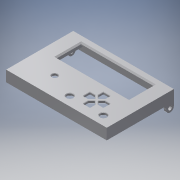
# Autodesk Inventor part: Interface Frame
Saved by Autodesk Inventor 2018 (Build 220112000, 112)
## iProperties
Created: 2018-03-12
Part Number: Interface Frame
Material: ABS Plastic
Document SubType Name: Modeling
Designer: Gabriel Smolnycki
Density: 1.06 g/cm^3
Appearance: Smooth - White
Author: Gabriel Smolnycki
Autodesk Inventor part; units mm, degrees
ref_plane "YZ Plane" through (0, 0, 0) normal (1, 0, 0) x (0, 1, 0)
ref_plane "XZ Plane" through (0, 0, 0) normal (0, 1, 0) x (-1, 0, 0)
sketch "Sketch1" plane through (0, 0, 0) normal (0, 0, 1) x (1, 0, 0)
  line L0 (-60, -40) -> (60, -40)
  line L1 (60, -40) -> (60, 40)
  line L2 (60, 40) -> (-60, 40)
  line L3 (-60, 40) -> (-60, -40)
  line L4 (-60, -40) -> (60, 40) construction
  line L5 (60, -40) -> (-60, 40) construction
  point P0 (0, 0)
  dimension "d0" = 120
  dimension "d1" = 80
  constraints: 12 end point, 2 midpoint, 2 parallel, 1 horizontal, 1 perpendicular
  measures "d0" distance of L2.end L1.end
  measures "d1" distance of L1.end L0.end
extrude "Extrusion1" add sketch "Sketch1" against normal blind 3
sketch "Sketch2" plane through (0, 0, 0) normal (0, 0, 1) x (1, 0, 0)
  line L0 (-43, 32.5) -> (43, 32.5)
  line L1 (43, 32.5) -> (43, 3.5)
  line L2 (43, 3.5) -> (-43, 3.5)
  line L3 (-43, 3.5) -> (-43, 32.5)
  line L4 (-43, 32.5) -> (43, 3.5) construction
  line L5 (43, 32.5) -> (-43, 3.5) construction
  point P0 (0, 0)
  point P1 (0, 18)
  dimension "d4" = 86
  dimension "d5" = 29
  dimension "d6" = 18
  constraints: 12 end point, 2 midpoint, 2 parallel, 1 horizontal, 1 perpendicular
  measures "d4" distance of L1.end L2.end
  measures "d5" distance of L0.end L1.end
  measures "d6" distance of point (0, 0) point (0, 18)
extrude "Extrusion2" cut sketch "Sketch2" against normal through all
chamfer "Chamfer1" distance 1.5 angle 45 4 edges at (-43, 18, 0) (0, 32.5, 0) (43, 18, 0) (0, 3.5, 0)
sketch "Sketch3" plane through (0, 0, 0) normal (0, 0, 1) x (1, 0, 0)
  line L0 (28.5, -29) -> (21.5, -29)
  line L1 (21, -28.5) -> (21, -23.2071)
  line L2 (29, -23.2071) -> (29, -28.5)
  line L3 (21.1464, -22.8536) -> (24.6464, -19.3536)
  line L4 (25.3536, -19.3536) -> (28.8536, -22.8536)
  arc A0 (21.1464, -22.8536) -> (21, -23.2071) centre (21.5, -23.2071) ccw
  arc A1 (21, -28.5) -> (21.5, -29) centre (21.5, -28.5) ccw
  arc A2 (28.5, -29) -> (29, -28.5) centre (28.5, -28.5) ccw
  arc A3 (29, -23.2071) -> (28.8536, -22.8536) centre (28.5, -23.2071) ccw
  arc A4 (25.3536, -19.3536) -> (24.6464, -19.3536) centre (25, -19.7071) ccw
  line L5 (60, -40) -> (60, 40) projected
  line L6 (-60, -40) -> (60, -40) projected
  line L7 (0, 0) -> (60, 0) construction
  line L8 (0, 0) -> (0, -40) construction
  line L9 (60, -40) -> (-60, -40) construction
  arc A5 (31.2071, -13) -> (30.8536, -13.1464) centre (31.2071, -13.5) ccw
  line L10 (31.2071, -13) -> (36.5, -13)
  arc A6 (27.3536, -16.6464) -> (27.3536, -17.3536) centre (27.7071, -17) ccw
  arc A7 (37, -13.5) -> (36.5, -13) centre (36.5, -13.5) ccw
  arc A8 (30.8536, -20.8536) -> (31.2071, -21) centre (31.2071, -20.5) ccw
  line L11 (30.8536, -20.8536) -> (27.3536, -17.3536)
  line L12 (36.5, -21) -> (31.2071, -21)
  arc A9 (36.5, -21) -> (37, -20.5) centre (36.5, -20.5) ccw
  line L13 (37, -13.5) -> (37, -20.5)
  line L14 (27.3536, -16.6464) -> (30.8536, -13.1464)
  arc A10 (21, -10.7929) -> (21.1464, -11.1464) centre (21.5, -10.7929) ccw
  line L15 (21, -10.7929) -> (21, -5.5)
  arc A11 (24.6464, -14.6464) -> (25.3536, -14.6464) centre (25, -14.2929) ccw
  arc A12 (21.5, -5) -> (21, -5.5) centre (21.5, -5.5) ccw
  arc A13 (28.8536, -11.1464) -> (29, -10.7929) centre (28.5, -10.7929) ccw
  line L16 (28.8536, -11.1464) -> (25.3536, -14.6464)
  line L17 (29, -5.5) -> (29, -10.7929)
  arc A14 (29, -5.5) -> (28.5, -5) centre (28.5, -5.5) ccw
  line L18 (21.5, -5) -> (28.5, -5)
  line L19 (24.6464, -14.6464) -> (21.1464, -11.1464)
  arc A15 (18.7929, -21) -> (19.1464, -20.8536) centre (18.7929, -20.5) ccw
  line L20 (18.7929, -21) -> (13.5, -21)
  arc A16 (22.6464, -17.3536) -> (22.6464, -16.6464) centre (22.2929, -17) ccw
  arc A17 (13, -20.5) -> (13.5, -21) centre (13.5, -20.5) ccw
  arc A18 (19.1464, -13.1464) -> (18.7929, -13) centre (18.7929, -13.5) ccw
  line L21 (19.1464, -13.1464) -> (22.6464, -16.6464)
  line L22 (13.5, -13) -> (18.7929, -13)
  arc A19 (13.5, -13) -> (13, -13.5) centre (13.5, -13.5) ccw
  line L23 (13, -20.5) -> (13, -13.5)
  line L24 (22.6464, -17.3536) -> (19.1464, -20.8536)
  circle A20 centre (45, -29) radius 4
  circle A21 centre (5, -29) radius 4
  circle A22 centre (-25, -17) radius 3.25
  point P0 (29, -29)
  point P1 (21, -29)
  point P2 (21, -23)
  point P3 (29, -23)
  point P4 (25, -19)
  point P5 (25, -17)
  point P6 (37, -13)
  point P7 (31, -13)
  point P8 (27, -17)
  point P9 (31, -21)
  point P10 (37, -21)
  point P11 (21, -5)
  point P12 (21, -11)
  point P13 (25, -15)
  point P14 (29, -11)
  point P15 (29, -5)
  point P16 (13, -21)
  point P17 (19, -21)
  point P18 (23, -17)
  point P19 (19, -13)
  point P20 (13, -13)
  dimension "d13" = 8
  dimension "d18" = 45
  dimension "d19" = 45
  dimension "d20" = 10
  dimension "d21" = 6
  dimension "d22" = 0.5
  dimension "d23" = 40
  dimension "d24" = 60
  dimension "d25" = 25
  dimension "d26" = 17
  dimension "d29" = 360
  dimension "d31" = 2
  dimension "d32" = 8
  dimension "d33" = 8
  dimension "d38" = 20
  dimension "d39" = 20
  dimension "d40" = 6.5
  dimension "d41" = 25
  dimension "d42" = 17
  dimension "d45" = 12
  dimension "d46" = 12
  constraints: 44 end point, 40 point on circle, 40 point on line, 23 centre point, 10 tangent, 4 equal radius, 2 midpoint, 2 perpendicular, 1 horizontal alignment, 1 vertical, 1 vertical alignment, 121 other
  measures "d13" distance of point (29, -29) point (21, -29)
  measures "d18" angle of L1 L3
  measures "d19" angle of L2 L4
  measures "d20" distance from line of L0 point (25, -19)
  measures "d21" distance of point (29, -29) point (29, -23)
  measures "d22" radius of A0
  measures "d23" distance of L7.start L8.end
  measures "d24" distance of L7.start L7.end
  measures "d25" distance from line of point (25, -17) L8
  measures "d26" distance from line of L7 point (25, -17)
  measures "d31" distance of point (25, -17) point (25, -19)
  measures "d32" diameter of A20
  measures "d33" diameter of A21
  measures "d38" horizontal distance of A20.centre point (25, -17)
  measures "d39" horizontal distance of A21.centre point (25, -17)
  measures "d40" diameter of A22
  measures "d41" distance from line of A22.centre L8
  measures "d42" vertical distance of L7.start A22.centre
  measures "d45" vertical distance of A21.centre point (25, -17)
  measures "d46" vertical distance of A20.centre point (25, -17)
extrude "Extrusion3" cut sketch "Sketch3" against normal through all
sketch "Sketch4" plane through (0, 0, -3) normal (0, 0, -1) x (-1, 0, 0)
  line L0 (60, -40) -> (60, 40) projected
  line L1 (-60, -40) -> (60, -40)
  line L2 (60, -40) -> (60, 40)
  line L3 (60, 40) -> (-60, 40)
  line L4 (-60, 40) -> (-60, -40)
  line L5 (-60, -40) -> (60, 40) construction
  line L6 (60, -40) -> (-60, 40) construction
  line L7 (-57, 37) -> (57, 37)
  line L8 (57, 37) -> (57, -37)
  line L9 (57, -37) -> (-57, -37)
  line L10 (-57, -37) -> (-57, 37)
  point P0 (0, 0)
  dimension "d47" = 3
  constraints: 20 end point, 4 parallel, 2 midpoint, 2 perpendicular, 1 horizontal, 3 other
  measures "d47" distance between parallel lines of L3 L7
extrude "Extrusion4" add sketch "Sketch4" along normal blind 10
sketch "Sketch5" plane through (60, -40, 0) normal (1, 0, 0) x (0, 0, -1)
  line L0 (13, 80) -> (13, 0) projected
  line L1 (0, 80) -> (13, 80) projected
  line L2 (0, 0) -> (0, 80) projected
  line L3 (13, 80) -> (13, 71)
  line L4 (13, 80) -> (17.5, 80)
  line L5 (17.5, 80) -> (17.5, 71) construction
  line L6 (17.5, 71) -> (13, 71)
  arc A0 (17.5, 71) -> (17.5, 80) centre (17.5, 75.5) ccw
  circle A1 centre (17.5, 75.5) radius 2.25
  point P0 (0, 40)
  dimension "d60" = 4.5
  dimension "d61" = 9
  dimension "d62" = 4.5
  dimension "d63" = 4.5
  constraints: 8 end point, 2 centre point, 2 perpendicular, 2 point on circle, 1 coincident, 1 horizontal, 1 point on line
  measures "d60" distance of L0.start L4.end
  measures "d61" distance of L0.start L3.end
  measures "d62" radius of A0
  measures "d63" diameter of A1
extrude "Extrusion5" add sketch "Sketch5" against normal up to surface (3 mm away)
mirror "Mirror1" about plane through (0, 0, 0) normal (1, 0, 0) of "Extrusion5"
fillet "Fillet2" radius 3 4 edges at (-57, 38.5, -13) (57, 38.5, -13) (58.5, 31, -13) (-58.5, 31, -13)
chamfer "Chamfer2" distance 0.5 angle 45 86 edges at (-28.25, -17, 0) (1, -29, 0) (21, -25.8536, 0) (21.0381, -23.0158, 0) (22.8964, -21.1036, 0) (25, -19.2071, 0) (27.1036, -21.1036, 0) (28.9619, -23.0158, 0) (29, -25.8536, 0) (28.8536, -28.8536, 0) (25, -29, 0) (21.1464, -28.8536, 0) (20.8964, -19.1036, 0) (18.9842, -20.9619, 0) (16.1464, -21, 0) (13.1464, -20.8536, 0) (13, -17, 0) (13.1464, -13.1464, 0) (16.1464, -13, 0) (18.9842, -13.0381, 0) (20.8964, -14.8964, 0) (22.7929, -17, 0) (25, -14.7929, 0) (22.8964, -12.8964, 0) (21.0381, -10.9842, 0) (21, -8.1464, 0) (21.1464, -5.1464, 0) (25, -5, 0) (28.8536, -5.1464, 0) (29, -8.1464, 0) (28.9619, -10.9842, 0) (27.1036, -12.8964, 0) (33.8536, -13, 0) (36.8536, -13.1464, 0) (37, -17, 0) (36.8536, -20.8536, 0) (33.8536, -21, 0) (31.0158, -20.9619, 0) (29.1036, -19.1036, 0) (27.2071, -17, 0) (29.1036, -14.8964, 0) (31.0158, -13.0381, 0) (41, -29, 0) (-28.25, -17, -3) (13, -17, -3) (13.1464, -20.8536, -3) (16.1464, -21, -3) (18.9842, -20.9619, -3) (20.8964, -19.1036, -3) (22.7929, -17, -3) (20.8964, -14.8964, -3) (18.9842, -13.0381, -3) (16.1464, -13, -3) (13.1464, -13.1464, -3) (1, -29, -3) (41, -29, -3) (25, -19.2071, -3) (22.8964, -21.1036, -3) (21.0381, -23.0158, -3) (21, -25.8536, -3) (21.1464, -28.8536, -3) (25, -29, -3) (28.8536, -28.8536, -3) (29, -25.8536, -3) (28.9619, -23.0158, -3) (27.1036, -21.1036, -3) (22.8964, -12.8964, -3) (25, -14.7929, -3) (27.1036, -12.8964, -3) (28.9619, -10.9842, -3) (29, -8.1464, -3) (28.8536, -5.1464, -3) (25, -5, -3) (21.1464, -5.1464, -3) (21, -8.1464, -3) (21.0381, -10.9842, -3) (29.1036, -14.8964, -3) (27.2071, -17, -3) (29.1036, -19.1036, -3) (31.0158, -20.9619, -3) (33.8536, -21, -3) (36.8536, -20.8536, -3) (37, -17, -3) (36.8536, -13.1464, -3) (33.8536, -13, -3) (31.0158, -13.0381, -3)
sketch "Sketch6" plane through (0, 0, -3) normal (0, 0, -1) x (-1, 0, 0)
  line L0 (-42.75, 3.75) -> (-46.75, 3.75) projected
  line L1 (-42.75, 4.25) -> (-42.75, 3.75) projected
  line L2 (42.75, 4.25) -> (-42.75, 4.25) projected
  line L3 (42.75, 3.75) -> (42.75, 4.25) projected
  line L4 (45.25, 3.75) -> (42.75, 3.75) projected
  line L5 (45.25, 5.5) -> (45.25, 3.75) projected
  line L6 (44.95, 5.5) -> (45.25, 5.5) projected
  arc A0 (44.95, 8) -> (44.95, 5.5) centre (44.95, 6.75) ccw projected
  line L7 (45.25, 8) -> (44.95, 8) projected
  line L8 (45.25, 31) -> (45.25, 8) projected
  line L9 (44.95, 31) -> (45.25, 31) projected
  arc A1 (44.95, 33.5) -> (44.95, 31) centre (44.95, 32.25) ccw projected
  line L10 (45.25, 33.5) -> (44.95, 33.5) projected
  line L11 (45.25, 35.25) -> (45.25, 33.5) projected
  line L12 (-46.75, 35.25) -> (45.25, 35.25) projected
  line L13 (-46.75, 33.5) -> (-46.75, 35.25) projected
  line L14 (-46.45, 33.5) -> (-46.75, 33.5) projected
  arc A2 (-46.45, 31) -> (-46.45, 33.5) centre (-46.45, 32.25) ccw projected
  line L15 (-46.75, 31) -> (-46.45, 31) projected
  line L16 (-46.75, 23.3) -> (-46.75, 31) projected
  line L17 (-43.75, 23.3) -> (-46.75, 23.3) projected
  arc A3 (-43.25, 22.8) -> (-43.75, 23.3) centre (-43.75, 22.8) ccw projected
  line L18 (-43.25, 13.3) -> (-43.25, 22.8) projected
  arc A4 (-43.75, 12.8) -> (-43.25, 13.3) centre (-43.75, 13.3) ccw projected
  line L19 (-46.75, 12.8) -> (-43.75, 12.8) projected
  line L20 (-46.75, 8) -> (-46.75, 12.8) projected
  line L21 (-46.45, 8) -> (-46.75, 8) projected
  arc A5 (-46.45, 5.5) -> (-46.45, 8) centre (-46.45, 6.75) ccw projected
  line L22 (-46.75, 5.5) -> (-46.45, 5.5) projected
  line L23 (-46.75, 3.75) -> (-46.75, 5.5) projected
  circle A6 centre (23.38, 33.75) radius 0.5 projected
  circle A7 centre (20.84, 33.75) radius 0.5 projected
  circle A8 centre (18.3, 33.75) radius 0.5 projected
  circle A9 centre (15.76, 33.75) radius 0.5 projected
  circle A10 centre (13.22, 33.75) radius 0.5 projected
  circle A11 centre (10.68, 33.75) radius 0.5 projected
  circle A12 centre (8.14, 33.75) radius 0.5 projected
  circle A13 centre (5.6, 33.75) radius 0.5 projected
  circle A14 centre (3.06, 33.75) radius 0.5 projected
  circle A15 centre (0.52, 33.75) radius 0.5 projected
  circle A16 centre (-2.02, 33.75) radius 0.5 projected
  circle A17 centre (-4.56, 33.75) radius 0.5 projected
  circle A18 centre (-7.1, 33.75) radius 0.5 projected
  circle A19 centre (-9.64, 33.75) radius 0.5 projected
  circle A20 centre (-12.18, 33.75) radius 0.5 projected
  circle A21 centre (-14.72, 33.75) radius 0.5 projected
  circle A22 centre (-17.26, 33.75) radius 0.5 projected
  circle A23 centre (-19.8, 33.75) radius 0.5 projected
  circle A24 centre (-22.34, 33.75) radius 0.5 projected
  circle A25 centre (-24.88, 33.75) radius 0.5 projected
  arc A26 (30.75, 32.3) -> (30.5, 32.55) centre (30.5, 32.3) ccw projected
  line L24 (30.75, 32.3) -> (30.75, 32) projected
  arc A27 (30.5, 31.75) -> (30.75, 32) centre (30.5, 32) ccw projected
  line L25 (30.5, 31.75) -> (26.5, 31.75) projected
  arc A28 (26.25, 32) -> (26.5, 31.75) centre (26.5, 32) ccw projected
  line L26 (26.25, 32) -> (26.25, 32.3) projected
  arc A29 (26.5, 32.55) -> (26.25, 32.3) centre (26.5, 32.3) ccw projected
  line L27 (26.5, 32.55) -> (30.5, 32.55) projected
  arc A30 (-27.75, 32.3) -> (-28, 32.55) centre (-28, 32.3) ccw projected
  line L28 (-27.75, 32.3) -> (-27.75, 32) projected
  arc A31 (-28, 31.75) -> (-27.75, 32) centre (-28, 32) ccw projected
  line L29 (-28, 31.75) -> (-32, 31.75) projected
  arc A32 (-32.25, 32) -> (-32, 31.75) centre (-32, 32) ccw projected
  line L30 (-32.25, 32) -> (-32.25, 32.3) projected
  arc A33 (-32, 32.55) -> (-32.25, 32.3) centre (-32, 32.3) ccw projected
  line L31 (-32, 32.55) -> (-28, 32.55) projected
  line L32 (-24.2929, -15) -> (-20.7929, -11.5) projected
  arc A34 (-25.7071, -15) -> (-24.2929, -15) centre (-25, -14.2929) ccw projected
  line L33 (-29.2071, -11.5) -> (-25.7071, -15) projected
  arc A35 (-29.5, -10.7929) -> (-29.2071, -11.5) centre (-28.5, -10.7929) ccw projected
  line L34 (-29.5, -5.5) -> (-29.5, -10.7929) projected
  arc A36 (-28.5, -4.5) -> (-29.5, -5.5) centre (-28.5, -5.5) ccw projected
  line L35 (-21.5, -4.5) -> (-28.5, -4.5) projected
  arc A37 (-20.5, -5.5) -> (-21.5, -4.5) centre (-21.5, -5.5) ccw projected
  line L36 (-20.5, -10.7929) -> (-20.5, -5.5) projected
  arc A38 (-20.7929, -11.5) -> (-20.5, -10.7929) centre (-21.5, -10.7929) ccw projected
  circle A39 centre (-45, -29) radius 4.5 projected
  line L37 (-12.5, -20.5) -> (-12.5, -13.5) projected
  arc A40 (-13.5, -21.5) -> (-12.5, -20.5) centre (-13.5, -20.5) ccw projected
  line L38 (-18.7929, -21.5) -> (-13.5, -21.5) projected
  arc A41 (-19.5, -21.2071) -> (-18.7929, -21.5) centre (-18.7929, -20.5) ccw projected
  line L39 (-23, -17.7071) -> (-19.5, -21.2071) projected
  arc A42 (-23, -16.2929) -> (-23, -17.7071) centre (-22.2929, -17) ccw projected
  line L40 (-19.5, -12.7929) -> (-23, -16.2929) projected
  arc A43 (-18.7929, -12.5) -> (-19.5, -12.7929) centre (-18.7929, -13.5) ccw projected
  line L41 (-13.5, -12.5) -> (-18.7929, -12.5) projected
  arc A44 (-12.5, -13.5) -> (-13.5, -12.5) centre (-13.5, -13.5) ccw projected
  line L42 (43, 32.5) -> (43, 3.5) projected
  line L43 (43, 3.5) -> (-43, 3.5) projected
  line L44 (-43, 3.5) -> (-43, 32.5) projected
  line L45 (-43, 32.5) -> (43, 32.5) projected
  line L46 (57, -37) -> (57, 37) projected
  line L47 (57, 37) -> (-57, 37) projected
  line L48 (-57, 37) -> (-57, -37) projected
  line L49 (-57, -37) -> (57, -37) projected
  circle A45 centre (25, -17) radius 3.75 projected
  circle A46 centre (-5, -29) radius 4.5 projected
  arc A47 (-24.2929, -19) -> (-25.7071, -19) centre (-25, -19.7071) ccw projected
  line L50 (-20.7929, -22.5) -> (-24.2929, -19) projected
  arc A48 (-20.5, -23.2071) -> (-20.7929, -22.5) centre (-21.5, -23.2071) ccw projected
  line L51 (-20.5, -28.5) -> (-20.5, -23.2071) projected
  arc A49 (-21.5, -29.5) -> (-20.5, -28.5) centre (-21.5, -28.5) ccw projected
  line L52 (-28.5, -29.5) -> (-21.5, -29.5) projected
  arc A50 (-29.5, -28.5) -> (-28.5, -29.5) centre (-28.5, -28.5) ccw projected
  line L53 (-29.5, -23.2071) -> (-29.5, -28.5) projected
  arc A51 (-29.2071, -22.5) -> (-29.5, -23.2071) centre (-28.5, -23.2071) ccw projected
  line L54 (-25.7071, -19) -> (-29.2071, -22.5) projected
  line L55 (-27, -16.2929) -> (-30.5, -12.7929) projected
  arc A52 (-27, -17.7071) -> (-27, -16.2929) centre (-27.7071, -17) ccw projected
  line L56 (-30.5, -21.2071) -> (-27, -17.7071) projected
  arc A53 (-31.2071, -21.5) -> (-30.5, -21.2071) centre (-31.2071, -20.5) ccw projected
  line L57 (-36.5, -21.5) -> (-31.2071, -21.5) projected
  arc A54 (-37.5, -20.5) -> (-36.5, -21.5) centre (-36.5, -20.5) ccw projected
  line L58 (-37.5, -13.5) -> (-37.5, -20.5) projected
  arc A55 (-36.5, -12.5) -> (-37.5, -13.5) centre (-36.5, -13.5) ccw projected
  line L59 (-31.2071, -12.5) -> (-36.5, -12.5) projected
  arc A56 (-30.5, -12.7929) -> (-31.2071, -12.5) centre (-31.2071, -13.5) ccw projected
  line L60 (-57, 3.75) -> (-44, 3.75)
  line L61 (-44, 3.75) -> (-44, 10.6358)
  line L62 (-44.2929, 11.3429) -> (-45.4571, 12.5071)
  line L63 (-57, 3.75) -> (-57, 37)
  line L64 (-57, 37) -> (-44, 37)
  line L65 (-45.75, 13.2142) -> (-45.75, 22.8858)
  line L66 (-45.4571, 23.5929) -> (-44.2929, 24.7571)
  line L67 (-45.75, 23.3) -> (-44.1036, 23.3) construction
  line L68 (-44, 37) -> (-44, 25.4642)
  circle A57 centre (-46.45, 32.25) radius 1.25
  circle A58 centre (-46.45, 6.75) radius 1.25
  arc A59 (-44.2929, 24.7571) -> (-44, 25.4642) centre (-45, 25.4642) ccw
  arc A60 (-45.4571, 23.5929) -> (-45.75, 22.8858) centre (-44.75, 22.8858) ccw
  arc A61 (-44, 10.6358) -> (-44.2929, 11.3429) centre (-45, 10.6358) ccw
  arc A62 (-45.75, 13.2142) -> (-45.4571, 12.5071) centre (-44.75, 13.2142) ccw
  line L69 (57, 37) -> (43, 37)
  line L70 (43, 37) -> (43, 3.75)
  line L71 (43, 3.75) -> (57, 3.75)
  point P0 (0, 0)
  point P1 (-44, 11.05)
  point P2 (-45.75, 12.8)
  point P3 (-44, 25.05)
  dimension "d71" = 13
  dimension "d73" = 135
  dimension "d74" = 1
  dimension "d75" = 45
  dimension "d76" = 1
  constraints: 24 end point, 17 point on line, 8 point on circle, 8 tangent, 4 centre point, 3 equal radius, 3 vertical alignment, 2 coincident, 2 collinear, 2 perpendicular, 2 vertical, 1 equal length, 1 horizontal, 4 other
  measures "d71" distance of L60.end L60.start
  measures "d73" angle of L62 L61
  measures "d74" distance from line of L20 point (-45.75, 12.8)
  measures "d75" angle of L67 L66
  measures "d76" radius of A59
extrude "Extrusion6" add sketch "Sketch6" along normal blind 2 contours L0 L23 L22 A5 L21 L20 L19 A62 L62 A61 L61 | L60 L48 L47 L68 L12 L13 L14 A57 L15 L16 L17 A60 L65 A62 L19 L20 L21 A58 L22 L23 | L42 L70 L12 L11 L10 A1 L9 L8 L7 A0 L6 L5 L4 | L47 L46 L71 L5 L6 A0 L7 L8 L9 A1 L10 L11 L12 L70 | L68 A59 L66 A60 L17 L16 L15 A2 L14 L13 L12
sketch "Sketch7" plane through (0, 0, -5) normal (0, 0, -1) x (-1, 0, 0)
  circle A0 centre (-46.45, 6.75) radius 1.25 projected
  circle A1 centre (-46.45, 32.25) radius 1.25 projected
  line L0 (-44, 3.75) -> (-44, 10.6358) projected
  arc A2 (-44, 10.6358) -> (-44.2929, 11.3429) centre (-45, 10.6358) ccw projected
  line L1 (-44.2929, 11.3429) -> (-45.4571, 12.5071) projected
  arc A3 (-45.75, 13.2142) -> (-45.4571, 12.5071) centre (-44.75, 13.2142) ccw projected
  line L2 (-45.75, 13.2142) -> (-45.75, 22.8858) projected
  arc A4 (-45.4571, 23.5929) -> (-45.75, 22.8858) centre (-44.75, 22.8858) ccw projected
  line L3 (-45.4571, 23.5929) -> (-44.2929, 24.7571) projected
  arc A5 (-44.2929, 24.7571) -> (-44, 25.4642) centre (-45, 25.4642) ccw projected
  line L4 (-44, 25.4642) -> (-44, 37) projected
  line L5 (-57, 37) -> (-44, 37) projected
  line L6 (-57, 3.75) -> (-57, 37) projected
  line L7 (-57, 3.75) -> (-44, 3.75) projected
  line L8 (43, 37) -> (43, 3.75) projected
  line L9 (43, 3.75) -> (57, 3.75) projected
  line L10 (57, 37) -> (57, 3.75) projected
  line L11 (43, 37) -> (57, 37) projected
  line L12 (-42.75, 3.75) -> (-46.75, 3.75) projected
  line L13 (-42.75, 4.25) -> (-42.75, 3.75) projected
  line L14 (42.75, 4.25) -> (-42.75, 4.25) projected
  line L15 (42.75, 3.75) -> (42.75, 4.25) projected
  line L16 (45.25, 3.75) -> (42.75, 3.75) projected
  line L17 (45.25, 5.5) -> (45.25, 3.75) projected
  line L18 (44.95, 5.5) -> (45.25, 5.5) projected
  arc A6 (44.95, 8) -> (44.95, 5.5) centre (44.95, 6.75) ccw projected
  line L19 (45.25, 8) -> (44.95, 8) projected
  line L20 (45.25, 31) -> (45.25, 8) projected
  line L21 (44.95, 31) -> (45.25, 31) projected
  arc A7 (44.95, 33.5) -> (44.95, 31) centre (44.95, 32.25) ccw projected
  line L22 (45.25, 33.5) -> (44.95, 33.5) projected
  line L23 (45.25, 35.25) -> (45.25, 33.5) projected
  line L24 (-46.75, 35.25) -> (45.25, 35.25) projected
  line L25 (-46.75, 33.5) -> (-46.75, 35.25) projected
  line L26 (-46.45, 33.5) -> (-46.75, 33.5) projected
  arc A8 (-46.45, 31) -> (-46.45, 33.5) centre (-46.45, 32.25) ccw projected
  line L27 (-46.75, 31) -> (-46.45, 31) projected
  line L28 (-46.75, 23.3) -> (-46.75, 31) projected
  line L29 (-43.75, 23.3) -> (-46.75, 23.3) projected
  arc A9 (-43.25, 22.8) -> (-43.75, 23.3) centre (-43.75, 22.8) ccw projected
  line L30 (-43.25, 13.3) -> (-43.25, 22.8) projected
  arc A10 (-43.75, 12.8) -> (-43.25, 13.3) centre (-43.75, 13.3) ccw projected
  line L31 (-46.75, 12.8) -> (-43.75, 12.8) projected
  line L32 (-46.75, 8) -> (-46.75, 12.8) projected
  line L33 (-46.45, 8) -> (-46.75, 8) projected
  arc A11 (-46.45, 5.5) -> (-46.45, 8) centre (-46.45, 6.75) ccw projected
  line L34 (-46.75, 5.5) -> (-46.45, 5.5) projected
  line L35 (-46.75, 3.75) -> (-46.75, 5.5) projected
  circle A12 centre (23.38, 33.75) radius 0.5 projected
  circle A13 centre (20.84, 33.75) radius 0.5 projected
  circle A14 centre (18.3, 33.75) radius 0.5 projected
  circle A15 centre (15.76, 33.75) radius 0.5 projected
  circle A16 centre (13.22, 33.75) radius 0.5 projected
  circle A17 centre (10.68, 33.75) radius 0.5 projected
  circle A18 centre (8.14, 33.75) radius 0.5 projected
  circle A19 centre (5.6, 33.75) radius 0.5 projected
  circle A20 centre (3.06, 33.75) radius 0.5 projected
  circle A21 centre (0.52, 33.75) radius 0.5 projected
  circle A22 centre (-2.02, 33.75) radius 0.5 projected
  circle A23 centre (-4.56, 33.75) radius 0.5 projected
  circle A24 centre (-7.1, 33.75) radius 0.5 projected
  circle A25 centre (-9.64, 33.75) radius 0.5 projected
  circle A26 centre (-12.18, 33.75) radius 0.5 projected
  circle A27 centre (-14.72, 33.75) radius 0.5 projected
  circle A28 centre (-17.26, 33.75) radius 0.5 projected
  circle A29 centre (-19.8, 33.75) radius 0.5 projected
  circle A30 centre (-22.34, 33.75) radius 0.5 projected
  circle A31 centre (-24.88, 33.75) radius 0.5 projected
  arc A32 (30.75, 32.3) -> (30.5, 32.55) centre (30.5, 32.3) ccw projected
  line L36 (30.75, 32.3) -> (30.75, 32) projected
  arc A33 (30.5, 31.75) -> (30.75, 32) centre (30.5, 32) ccw projected
  line L37 (30.5, 31.75) -> (26.5, 31.75) projected
  arc A34 (26.25, 32) -> (26.5, 31.75) centre (26.5, 32) ccw projected
  line L38 (26.25, 32) -> (26.25, 32.3) projected
  arc A35 (26.5, 32.55) -> (26.25, 32.3) centre (26.5, 32.3) ccw projected
  line L39 (26.5, 32.55) -> (30.5, 32.55) projected
  arc A36 (-27.75, 32.3) -> (-28, 32.55) centre (-28, 32.3) ccw projected
  line L40 (-27.75, 32.3) -> (-27.75, 32) projected
  arc A37 (-28, 31.75) -> (-27.75, 32) centre (-28, 32) ccw projected
  line L41 (-28, 31.75) -> (-32, 31.75) projected
  arc A38 (-32.25, 32) -> (-32, 31.75) centre (-32, 32) ccw projected
  line L42 (-32.25, 32) -> (-32.25, 32.3) projected
  arc A39 (-32, 32.55) -> (-32.25, 32.3) centre (-32, 32.3) ccw projected
  line L43 (-32, 32.55) -> (-28, 32.55) projected
  line L44 (-57, 35.25) -> (-47, 35.25)
  line L45 (-44, 3.75) -> (-57, 3.75) projected
  line L46 (-57, 3.75) -> (-57, -37) projected
  line L47 (-57, 3.75) -> (-47, 3.75)
  line L48 (-57, 3.75) -> (-57, 35.25)
  circle A40 centre (-46.45, 32.25) radius 1.25 projected
  arc A41 (-47, 33.3725) -> (-47, 31.1275) centre (-46.45, 32.25) ccw
  circle A42 centre (-46.45, 6.75) radius 1.25 projected
  arc A43 (-47, 7.8725) -> (-47, 5.6275) centre (-46.45, 6.75) ccw
  line L49 (-47, 5.6275) -> (-47, 3.75)
  line L50 (-47, 35.25) -> (-47, 33.3725)
  line L51 (-47, 31.1275) -> (-47, 7.8725)
  line L52 (57, 35.25) -> (45.5, 35.25)
  line L53 (57, 3.75) -> (43, 3.75) projected
  line L54 (57, 3.75) -> (45.5, 3.75)
  line L55 (57, 3.75) -> (57, 35.25)
  arc A44 (45.5, 31.1275) -> (45.5, 33.3725) centre (44.95, 32.25) ccw
  arc A45 (45.5, 5.6275) -> (45.5, 7.8725) centre (44.95, 6.75) ccw
  line L56 (45.5, 5.6275) -> (45.5, 3.75)
  line L57 (45.5, 35.25) -> (45.5, 33.3725)
  line L58 (45.5, 31.1275) -> (45.5, 7.8725)
  line L59 (43, 37) -> (-44, 37) projected
  line L60 (-44, 37) -> (-44, 35.5)
  line L61 (-44, 37) -> (-44, 25.4642) projected
  line L62 (-44, 35.5) -> (-47, 35.5)
  line L63 (-47, 35.5) -> (-47, 35.25)
  line L64 (-44, 37) -> (-57, 37)
  line L65 (-57, 37) -> (-57, 35.25)
  line L66 (43, 37) -> (43, 35.5)
  line L67 (43, 32.5) -> (43, 37) projected
  line L68 (43, 35.5) -> (45.5, 35.5)
  line L69 (45.5, 35.5) -> (45.5, 35.25)
  line L70 (57, 35.25) -> (57, 37)
  line L71 (43, 37) -> (57, 37)
  point P0 (0, 0)
  dimension "d80" = 10.25
  dimension "d81" = 10
  dimension "d82" = 10
  dimension "d83" = 10
  dimension "d84" = 11.75
  dimension "d85" = 11.5
  dimension "d86" = 1.25
  dimension "d87" = 1.25
  dimension "d88" = 11.5
  dimension "d89" = 11.5
  dimension "d92" = 1.75
  dimension "d93" = 1.5
  dimension "d94" = 1.5
  constraints: 44 end point, 12 perpendicular, 12 point on circle, 7 point on line, 6 collinear, 4 centre point, 4 coincident, 2 horizontal
  measures "d80" distance between parallel lines of L6 L25
  measures "d81" distance of L44.start L44.end
  measures "d82" distance between parallel lines of L48 L51
  measures "d83" distance between parallel lines of L48 L49
  measures "d84" distance between parallel lines of L10 L23
  measures "d85" distance of L52.start L52.end
  measures "d86" radius of A44
  measures "d87" radius of A45
  measures "d88" distance between parallel lines of L10 L58
  measures "d89" distance between parallel lines of L10 L56
  measures "d92" distance between parallel lines of L59 L24
  measures "d93" distance of L4.end L60.end
  measures "d94" distance of L8.start L66.end
ref_plane "Work Plane1" through (-45.25, 3.75, -6) normal (0, 0, -1) x (0, 1, 0)
extrude "Extrusion7" add sketch "Sketch7" along normal up to surface (1 mm away) contours A0 L49 L7 L6 L44 L50 A1 L51 | L44 L6 L5 L4 L62 L63 | L11 L10 L52 L69 L68 L8 | L10 L9 L56 A45 L58 A44 L57 L52
equation "\"d39\" = d38"
equation "\"d41\" = d25"
equation "\"d42\" = d26"
equation "\"d62\" = 0.5 * d61"
equation "\"d63\" = d62"
body "Solid1"
